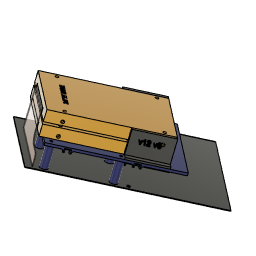
IDE Drive Bench Large and Models v12 v7 (Autodesk Fusion 360 design; units mm, degrees)
Autodesk Fusion 360 part; units mm, degrees
note: some values were not read from the file. Set by a fixed rule: which sketch regions a step uses.
sketch "Sketch1" plane through (0, 0, 0) normal (0, 1, 0) x (1, 0, 0)
  line L0 (0, 0) -> (-110, 0)
  line L1 (-110, 0) -> (-110, -88)
  line L2 (-110, -88) -> (0, -88)
  line L3 (0, -88) -> (0, 0)
  dimension "d1" = 110
  dimension "d2" = 88
  constraint horizontal L0
  constraint vertical L1
  constraint horizontal L2
  constraint vertical L3
  constraint coincident L0.start L3.end
  measures "d1" distance of L0.start L0.end
  measures "d2" distance of L0.start L2.end
extrude "Extrude1" add sketch "Sketch1" along normal blind 2.25 makes body 1
sketch "Pillars to JM003A" plane through (0, 2.25, 0) normal (0, 1, 0) x (-1, 0, 0)
  line L0 (0, 88) -> (0, 0)
  line L1 (0, 0) -> (110, 0)
  line L2 (110, 0) -> (110, 88)
  line L3 (110, 88) -> (0, 88)
  line L4 (5.6675, 45.75) -> (59.1675, 45.75)
  line L5 (59.1675, 45.75) -> (59.1675, 82.75)
  line L6 (59.1675, 82.75) -> (5.6675, 82.75)
  line L7 (5.6675, 82.75) -> (5.6675, 45.75)
  circle A0 centre (59.1675, 45.75) radius 1.25
  circle A1 centre (59.1675, 82.75) radius 1.25
  circle A2 centre (5.6675, 82.75) radius 1.25
  circle A3 centre (5.6675, 45.75) radius 1.25
  circle A4 centre (59.1675, 45.75) radius 3.5
  circle A5 centre (5.6675, 45.75) radius 3.5
  circle A6 centre (59.1675, 82.75) radius 3.5
  circle A7 centre (5.6675, 82.75) radius 3.5
  dimension "d5" = 53.5
  dimension "d6" = 37
  dimension "d7" = 2.5
  dimension "d8" = 2.5
  dimension "d9" = 2.5
  dimension "d10" = 2.5
  dimension "d11" = 7
  dimension "d12" = 7
  dimension "d13" = 7
  dimension "d14" = 7
  dimension "d184" = 5.25
  constraint horizontal L4
  constraint vertical L5
  constraint horizontal L6
  constraint vertical L7
  constraint coincident L4.end L5.start
  constraint coincident L5.end L6.start
  constraint coincident L6.end L7.start
  constraint coincident L4.start L7.end
  constraint concentric A0 A4
  constraint concentric A3 A5
  constraint concentric A1 A6
  constraint concentric A2 A7
  measures "d5" distance of L4.start L4.end
  measures "d6" distance of L4.start L6.end
  measures "d7" diameter of A0
  measures "d8" diameter of A1
  measures "d9" diameter of A2
  measures "d10" diameter of A3
  measures "d11" diameter of A4
  measures "d12" diameter of A5
  measures "d13" diameter of A6
  measures "d14" diameter of A7
  measures "d184" distance of L3 L6.end
extrude "Extrude2" add sketch "Pillars to JM003A" along normal blind 19.5 contours L4 L7 A3 A5 | L4 L7 A3 A5 | L4 L5 A0 A4 | L4 L5 A0 A4 | L6 L7 A2 A7 | L6 L7 A2 A7 | L5 L6 A1 A6 | L5 L6 A1 A6 bodies 1
sketch "Sketch3" plane through (0, 2.25, 0) normal (0, 1, 0) x (-1, 0, 0)
  circle A0 centre (59.1675, 45.75) radius 3.5
  circle A1 centre (59.1675, 82.75) radius 3.5
  line L0 (0, 88) -> (0, 0)
  line L1 (0, 0) -> (110, 0)
  line L2 (110, 0) -> (110, 88)
  line L3 (110, 88) -> (0, 88)
  circle A2 centre (5.6675, 82.75) radius 3.5
  circle A3 centre (5.6675, 45.75) radius 3.5
  line L4 (75, 0) -> (73.5, 0)
  line L5 (73.5, 0) -> (73.5, 2.5)
  line L6 (73.5, 2.5) -> (75, 2.5)
  line L7 (75, 2.5) -> (75, 0)
  line L8 (14.9953, 0) -> (16.4953, 0)
  line L9 (16.4953, 0) -> (16.4953, 2.5)
  line L10 (16.4953, 2.5) -> (14.9953, 2.5)
  line L11 (14.9953, 2.5) -> (14.9953, 0)
  line L12 (75, 88) -> (73.5, 88)
  line L13 (73.5, 88) -> (73.5, 85.5)
  line L14 (73.5, 85.5) -> (75, 85.5)
  line L15 (75, 85.5) -> (75, 88)
  line L16 (14.9794, 88) -> (16.4794, 88)
  line L17 (16.4794, 88) -> (16.4794, 85.5)
  line L18 (16.4794, 85.5) -> (14.9794, 85.5)
  line L19 (14.9794, 85.5) -> (14.9794, 88)
  line L20 (70, 0) -> (68.5, 0)
  line L21 (68.5, 0) -> (68.5, 2.5)
  line L22 (68.5, 2.5) -> (70, 2.5)
  line L23 (70, 2.5) -> (70, 0)
  line L24 (19.9953, 0) -> (21.4953, 0)
  line L25 (21.4953, 0) -> (21.4953, 2.5)
  line L26 (21.4953, 2.5) -> (19.9953, 2.5)
  line L27 (19.9953, 2.5) -> (19.9953, 0)
  line L28 (70, 88) -> (68.5, 88)
  line L29 (68.5, 88) -> (68.5, 85.5)
  line L30 (68.5, 85.5) -> (70, 85.5)
  line L31 (70, 85.5) -> (70, 88)
  line L32 (19.9794, 88) -> (21.4794, 88)
  line L33 (21.4794, 88) -> (21.4794, 85.5)
  line L34 (21.4794, 85.5) -> (19.9794, 85.5)
  line L35 (19.9794, 85.5) -> (19.9794, 88)
  dimension "d17" = 1.5
  dimension "d18" = 2.5
  dimension "d19" = 1.5
  dimension "d20" = 2.5
  dimension "d21" = 1.5
  dimension "d22" = 2.5
  dimension "d23" = 1.5
  dimension "d24" = 2.5
  dimension "d25" = 1.5
  dimension "d26" = 2.5
  dimension "d27" = 3.5
  dimension "d28" = 1.5
  dimension "d29" = 2.5
  dimension "d30" = 3.5
  dimension "d31" = 1.5
  dimension "d32" = 2.5
  dimension "d33" = 3.5
  dimension "d34" = 1.5
  dimension "d35" = 2.5
  dimension "d36" = 3.5
  dimension "d185" = 35
  dimension "d186" = 35
  constraint horizontal L4
  constraint vertical L5
  constraint horizontal L6
  constraint vertical L7
  constraint coincident L1 L4.start
  constraint horizontal L8
  constraint vertical L9
  constraint horizontal L10
  constraint vertical L11
  constraint coincident L1 L8.start
  constraint horizontal L12
  constraint vertical L13
  constraint horizontal L14
  constraint vertical L15
  constraint coincident L3 L12.start
  constraint horizontal L16
  constraint vertical L17
  constraint horizontal L18
  constraint vertical L19
  constraint coincident L3 L16.start
  constraint horizontal L20
  constraint vertical L21
  constraint horizontal L22
  constraint vertical L23
  constraint coincident L1 L20.start
  constraint horizontal L24
  constraint vertical L25
  constraint horizontal L26
  constraint vertical L27
  constraint coincident L1 L24.start
  constraint horizontal L28
  constraint vertical L29
  constraint horizontal L30
  constraint vertical L31
  constraint coincident L3 L28.start
  constraint horizontal L32
  constraint vertical L33
  constraint horizontal L34
  constraint vertical L35
  constraint coincident L3 L32.start
  measures "d17" distance of L4.start L4.end
  measures "d18" distance of L4.start L6.end
  measures "d19" distance of L8.start L8.end
  measures "d20" distance of L8.start L10.end
  measures "d21" distance of L12.start L12.end
  measures "d22" distance of L12.start L14.end
  measures "d23" distance of L16.start L16.end
  measures "d24" distance of L16.start L18.end
  measures "d25" distance of L20.start L20.end
  measures "d26" distance of L20.start L22.end
  measures "d27" distance of L5 L23
  measures "d28" distance of L24.start L24.end
  measures "d29" distance of L24.start L26.end
  measures "d30" distance of L9 L27
  measures "d31" distance of L28.start L28.end
  measures "d32" distance of L28.start L30.end
  measures "d33" distance of L13 L31
  measures "d34" distance of L32.start L32.end
  measures "d35" distance of L32.start L34.end
  measures "d36" distance of L17 L35
  measures "d185" distance of L2 L15
  measures "d186" distance of L2 L7
extrude "Extrude3" add sketch "Sketch3" along normal blind 2.5 contours L3 L16 L17 L18 L19 | L3 L32 L33 L34 L35 bodies 1
extrude "Extrude4" add sketch "Sketch3" along normal blind 2.5 contours L3 L28 L29 L30 L31 | L3 L12 L13 L14 L15 bodies 1
extrude "Extrude5" add sketch "Sketch3" along normal blind 2.5 contours L1 L20 L21 L22 L23 | L1 L4 L5 L6 L7 bodies 1
extrude "Extrude6" add sketch "Sketch3" along normal blind 2.5 contours L1 L8 L9 L10 L11 | L1 L24 L25 L26 L27 bodies 1
fillet "Fillet1" radius 1 2 edges at (-73.5, 3.5, 88) (-70, 3.5, 88) on bodies 1
fillet "Fillet2" radius 1 2 edges at (-19.9794, 3.5, 88) (-16.4794, 3.5, 88) on bodies 1
fillet "Fillet3" radius 1 2 edges at (-16.4953, 3.5, 0) (-19.9953, 3.5, 0) on bodies 1
fillet "Fillet4" radius 1 2 edges at (-70, 3.5, 0) (-73.5, 3.5, 0) on bodies 1
fillet "Fillet5" radius 2 4 edges at (-75, 2.25, 86.75) (-75, 2.25, 1.25) (-21.4953, 2.25, 1.25) (-21.4794, 2.25, 86.75) on bodies 1
fillet "Fillet6" radius 2 4 edges at (-21.7453, 2.25, 2.5) (-75.25, 2.25, 2.5) (-75.25, 2.25, 85.5) (-21.7294, 2.25, 85.5) on bodies 1
fillet "Fillet7" radius 2 4 edges at (-68.5, 2.25, 86.75) (-68.5, 2.25, 1.25) (-14.9794, 2.25, 86.75) (-14.9953, 2.25, 1.25) on bodies 1
fillet "Fillet8" radius 2 4 edges at (-68.25, 2.25, 2.5) (-14.7453, 2.25, 2.5) (-14.7294, 2.25, 85.5) (-68.25, 2.25, 85.5) on bodies 1
fillet "Fillet10" radius 1 4 edges at (-71.75, 2.25, 0) (-18.2453, 2.25, 0) (-18.2294, 2.25, 88) (-71.75, 2.25, 88) on bodies 1
sketch "Version String" plane through (0, 2.25, 0) normal (0, 1, 0) x (-1, 0, 0)
  line L0 (73.5, 87) -> (70, 87)
  line L1 (70, 87) -> (70, 83.5)
  line L2 (66.5, 83.5) -> (66.5, 88)
  line L3 (66.5, 88) -> (23.4794, 88)
  line L4 (23.4794, 88) -> (23.4794, 83.5)
  line L5 (23.4794, 83.5) -> (19.9794, 83.5)
  line L6 (19.9794, 83.5) -> (19.9794, 87)
  line L7 (19.9794, 87) -> (16.4794, 87)
  line L8 (16.4794, 87) -> (16.4794, 83.5)
  line L9 (16.4794, 83.5) -> (12.9794, 83.5)
  line L10 (12.9794, 83.5) -> (12.9794, 88)
  line L11 (12.9794, 88) -> (0, 88)
  line L12 (0, 88) -> (0, 0)
  line L13 (0, 0) -> (12.9953, 0)
  line L14 (12.9953, 0) -> (12.9953, 4.5)
  line L15 (12.9953, 4.5) -> (16.4953, 4.5)
  line L16 (16.4953, 4.5) -> (16.4953, 1)
  line L17 (16.4953, 1) -> (19.9953, 1)
  line L18 (19.9953, 1) -> (19.9953, 4.5)
  line L19 (19.9953, 4.5) -> (23.4953, 4.5)
  line L20 (23.4953, 4.5) -> (23.4953, 0)
  line L21 (23.4953, 0) -> (66.5, 0)
  line L22 (66.5, 0) -> (66.5, 4.5)
  line L23 (66.5, 4.5) -> (70, 4.5)
  line L24 (70, 4.5) -> (70, 1)
  line L25 (70, 1) -> (73.5, 1)
  line L26 (73.5, 1) -> (73.5, 4.5)
  line L27 (73.5, 4.5) -> (77, 4.5)
  line L28 (77, 4.5) -> (77, 0)
  line L29 (77, 0) -> (110, 0)
  line L30 (110, 0) -> (110, 88)
  line L31 (110, 88) -> (77, 88)
  line L32 (77, 88) -> (77, 83.5)
  line L33 (77, 83.5) -> (73.5, 83.5)
  line L34 (73.5, 83.5) -> (73.5, 87)
  line L35 (63.5441, 32.548) -> (63.5441, 16.8859) construction
  line L36 (63.5441, 16.8859) -> (69.5441, 16.8859) construction
  line L37 (69.5441, 16.8859) -> (69.5441, 32.548) construction
  line L38 (69.5441, 32.548) -> (63.5441, 32.548) construction
  circle A0 centre (5.6675, 82.75) radius 3.5
  circle A1 centre (5.6675, 45.75) radius 3.5
  circle A2 centre (59.1675, 45.75) radius 3.5
  line L39 (70, 83.5) -> (66.5, 83.5)
  circle A3 centre (59.1675, 82.75) radius 3.5
  text T0 "v12v3" font "Arial" height 6 align ink ink in box 0 x 0 at (63.5641, 32.538) x (0, -1) y (1, 0) spacing 1 height is em
  constraint perpendicular L35 L36
  constraint parallel L35 L37
  constraint parallel L36 L38
extrude "Extrude7" add sketch "Version String" along normal blind 1 text T0 bodies 1
fillet "Fillet11" radius 1 4 edges at (-4.5021, 21.75, 46.202) (-4.5021, 21.75, 83.202) (-58.0021, 21.75, 83.202) (-58.0021, 21.75, 46.202) on bodies 1
ref_plane "WorkPlane1" through (-55, -10, 44) normal (0, 1, 0) x (1, 0, 0)
sketch "Sketch5" plane through (0, 0, 0) normal (0, 1, 0) x (1, 0, 0)
sketch "Sketch6" plane through (-42.5, -10, 44) normal (0, 1, 0) x (1, 0, 0)
  line L0 (40.0162, -34.9034) -> (-59.9838, -34.9034)
  line L1 (-59.9838, -34.9034) -> (-59.9838, 35.0966)
  line L2 (-59.9838, 35.0966) -> (40.0162, 35.0966)
  line L3 (40.0162, 35.0966) -> (40.0162, -34.9034)
  dimension "d59" = 100
  dimension "d60" = 70
  constraint horizontal L0
  constraint vertical L1
  constraint horizontal L2
  constraint vertical L3
  measures "d59" distance of L0.start L0.end
  measures "d60" distance of L0.start L2.end
extrude "Extrude8" add sketch "Sketch6" against normal blind 10 separate body makes body 2
sketch "Sketch7" plane through (0, -20, 0) normal (0, -1, 0) x (1, 0, 0)
  line L0 (-102.4838, 8.9034) -> (-2.4838, 8.9034)
  line L1 (-2.4838, 8.9034) -> (-2.4838, 78.9034)
  line L2 (-2.4838, 78.9034) -> (-102.4838, 78.9034)
  line L3 (-102.4838, 78.9034) -> (-102.4838, 8.9034)
  line L4 (-20.7994, 59.6561) -> (-20.7994, 27.1781) construction
  line L5 (-20.7994, 27.1781) -> (-15.7994, 27.1781) construction
  line L6 (-15.7994, 27.1781) -> (-15.7994, 59.6561) construction
  line L7 (-15.7994, 59.6561) -> (-20.7994, 59.6561) construction
  text T0 "2.5\" FF DRIVE" font "Arial" height 5 align ink ink in box 0 x 0 at (-20.7794, 59.6461) x (0, -1) y (1, 0) spacing 1 height is em
  constraint perpendicular L4 L5
  constraint parallel L4 L6
  constraint parallel L5 L7
extrude "Extrude9" cut sketch "Sketch7" against normal blind 1 text T0 bodies 2
sketch "Sketch8" plane through (0, 0, 78.9034) normal (0, 0, 1) x (1, 0, 0)
  line L0 (-2.4838, -10) -> (-102.4838, -10)
  line L1 (-102.4838, -10) -> (-102.4838, -20)
  line L2 (-102.4838, -20) -> (-2.4838, -20)
  line L3 (-2.4838, -20) -> (-2.4838, -10)
  circle A0 centre (-16.4838, -13) radius 1.5
  line L4 (-2.4838, -10) -> (-102.4838, -10)
  circle A1 centre (-93.0838, -12.9925) radius 1.5
  dimension "d65" = 3
  dimension "d66" = 14
  dimension "d67" = 3
  dimension "d68" = 3
  dimension "d69" = 90.6
  measures "d65" diameter of A0
  measures "d66" distance of L3 A0.centre
  measures "d67" distance of A0.centre L4
  measures "d68" diameter of A1
  measures "d69" distance of L3 A1.centre
extrude "Extrude10" cut sketch "Sketch8" against normal blind 70 contours A1 bodies 2
extrude "Extrude11" cut sketch "Sketch8" against normal blind 70 contours A0 bodies 2
sketch "Sketch9" plane through (0, -10, 0) normal (0, 1, 0) x (-1, 0, 0)
  line L0 (2.4838, 8.9034) -> (102.4838, 8.9034)
  line L1 (102.4838, 8.9034) -> (102.4838, 78.9034)
  line L2 (102.4838, 78.9034) -> (2.4838, 78.9034)
  line L3 (2.4838, 78.9034) -> (2.4838, 8.9034)
  circle A0 centre (16.4838, 74.8334) radius 1.5
  line L4 (2.4838, 78.9034) -> (102.4838, 78.9034)
  circle A1 centre (16.4838, 12.9734) radius 1.5
  circle A2 centre (93.0838, 74.8334) radius 1.5
  circle A3 centre (93.0838, 12.9734) radius 1.5
  dimension "d74" = 3
  dimension "d75" = 14
  dimension "d76" = 4.07
  dimension "d77" = 3
  dimension "d78" = 14
  dimension "d79" = 4.07
  dimension "d80" = 3
  dimension "d81" = 90.6
  dimension "d82" = 4.07
  dimension "d83" = 3
  dimension "d84" = 90.6
  dimension "d85" = 4.07
  measures "d74" diameter of A0
  measures "d75" distance of L3 A0.centre
  measures "d76" distance of A0.centre L4
  measures "d77" diameter of A1
  measures "d78" distance of L3 A1.centre
  measures "d79" distance of L0 A1.centre
  measures "d80" diameter of A2
  measures "d81" distance of L3 A2.centre
  measures "d82" distance of L2 A2.centre
  measures "d83" diameter of A3
  measures "d84" distance of L3 A3.centre
  measures "d85" distance of L0 A3.centre
extrude "Extrude12" cut sketch "Sketch9" against normal blind 10 contours A0 | A1 | A2 | A3 bodies 2
sketch "IDE Connector Recess" plane through (-2.4838, 0, 0) normal (1, 0, 0) x (0, 0, -1)
  line L0 (-8.9034, -10) -> (-78.9034, -10)
  line L1 (-78.9034, -10) -> (-78.9034, -20)
  line L2 (-78.9034, -20) -> (-8.9034, -20)
  line L3 (-8.9034, -20) -> (-8.9034, -10)
  line L4 (-62.9034, -10) -> (-18.9034, -10)
  line L5 (-18.9034, -10) -> (-18.9034, -14)
  line L6 (-18.9034, -14) -> (-62.9034, -14)
  line L7 (-62.9034, -14) -> (-62.9034, -10)
  dimension "d100" = 44
  dimension "d101" = 4
  dimension "d174" = 16
  dimension "d175" = 10
  constraint horizontal L4
  constraint vertical L5
  constraint horizontal L6
  constraint vertical L7
  constraint coincident L0 L4.start
  measures "d100" distance of L4.start L4.end
  measures "d101" distance of L4.start L6.end
  measures "d174" distance of L1 L7
  measures "d175" distance of L3 L5
extrude "Extrude13" cut sketch "IDE Connector Recess" against normal blind 4 contours L0 L4 L5 L6 L7 bodies 2
sketch "Sketch11" plane through (0, 0, 0) normal (0, -1, 0) x (1, 0, 0)
  line L0 (0, 0) -> (0, 88)
  line L1 (0, 88) -> (-110, 88)
  line L2 (-110, 88) -> (-110, 0)
  line L3 (-110, 0) -> (0, 0)
  line L4 (-0.0039, 28.8454) -> (-4.0039, 28.8454)
  line L5 (-4.0039, 28.8454) -> (-4.0039, 72.8454)
  line L6 (-4.0039, 72.8454) -> (-0.0039, 72.8454)
  line L7 (-0.0039, 72.8454) -> (-0.0039, 28.8454)
  dimension "d104" = 4
  dimension "d105" = 44
  constraint horizontal L4
  constraint vertical L5
  constraint horizontal L6
  constraint vertical L7
  measures "d104" distance of L4.start L4.end
  measures "d105" distance of L4.start L6.end
sketch "Sketch12" plane through (0, 0, 0) normal (0, 1, 0) x (1, 0, 0)
  line L0 (15.0376, -24.9871) -> (11.0376, -24.9871)
  line L1 (11.0376, -24.9871) -> (11.0376, -68.9871)
  line L2 (11.0376, -68.9871) -> (15.0376, -68.9871)
  line L3 (15.0376, -68.9871) -> (15.0376, -24.9871)
  dimension "d106" = 4
  dimension "d107" = 44
  constraint horizontal L0
  constraint vertical L1
  constraint horizontal L2
  constraint vertical L3
  measures "d106" distance of L0.start L0.end
  measures "d107" distance of L0.start L2.end
extrude "Extrude14" add sketch "Sketch12" along normal blind 4 separate body makes body 3
move_body "Move1" bodies 3 to x (1, 0, 0) y (0, 1, 0) z (0, 0, 1) at (-17.4241, -4.5506, 3.881)
copy_body "CopyPasteBodies1" bodies 3 makes body 4
move_body "Move2" bodies 4 to x (1, 0, 0) y (0, 1, 0) z (0, 0, 1) at (0, -5.6283, 0)
move_body "Move3" bodies 2 to x (1, 0, 0) y (0, 1, 0) z (0, 0, 1) at (0, -7.1851, -0.2395)
ref_plane "WorkPlane2" through (-5.6675, 31.75, 45.75) normal (0, 1, 0) x (-1, 0, 0)
sketch "JM003A Card Outlone" plane through (-5.6675, 31.75, 44.8014) normal (0, 1, 0) x (1, 0, 0)
  line L0 (16.3291, -49.8685) -> (-141.6709, -49.8685)
  line L1 (-141.6709, -49.8685) -> (-141.6709, 40.1315)
  line L2 (-141.6709, 40.1315) -> (16.3291, 40.1315)
  line L3 (16.3291, 40.1315) -> (16.3291, -49.8685)
  line L4 (-45.6709, 40.1315) -> (-141.6709, 40.1315)
  line L5 (-141.6709, 40.1315) -> (-141.6709, 73.6737)
  line L6 (-141.6709, 73.6737) -> (-45.6709, 73.6737)
  line L7 (-45.6709, 73.6737) -> (-45.6709, 40.1315)
  dimension "d111" = 158
  dimension "d112" = 90
  dimension "d113" = 96
  dimension "d114" = 62
  constraint horizontal L0
  constraint vertical L1
  constraint horizontal L2
  constraint vertical L3
  constraint horizontal L4
  constraint vertical L5
  constraint horizontal L6
  constraint vertical L7
  constraint coincident L2 L4.start
  measures "d111" distance of L0.start L0.end
  measures "d112" distance of L0.start L2.end
  measures "d113" distance of L5.end L6.end
  measures "d114" distance of L3 L7
extrude "Extrude15" add sketch "JM003A Card Outlone" along normal blind 0.6 separate body makes body 5
sketch "Sketch15" plane through (0, 32.35, 0) normal (0, 1, 0) x (-1, 0, 0)
  line L0 (51.3384, -28.8723) -> (147.3384, -28.8723)
  line L1 (147.3384, -28.8723) -> (147.3384, 94.6698)
  line L2 (147.3384, 94.6698) -> (-10.6616, 94.6698)
  line L3 (-10.6616, 94.6698) -> (-10.6616, 4.6698)
  line L4 (-10.6616, 4.6698) -> (51.3384, 4.6698)
  line L5 (51.3384, 4.6698) -> (51.3384, -28.8723)
  circle A0 centre (4.3384, 89.6698) radius 1.5
  circle A1 centre (4.3384, 50.6698) radius 1.5
  circle A2 centre (69.3384, 50.6698) radius 1.5
  circle A3 centre (69.3384, 89.6698) radius 1.5
  dimension "d121" = 3
  dimension "d122" = 15
  dimension "d123" = 5
  dimension "d124" = 3
  dimension "d125" = 15
  dimension "d126" = 39
  dimension "d127" = 3
  dimension "d128" = 80
  dimension "d129" = 3
  dimension "d130" = 5
  dimension "d131" = 39
  dimension "d134" = 80
  measures "d121" diameter of A0
  measures "d122" distance of L3 A0.centre
  measures "d123" distance of L2 A0.centre
  measures "d124" diameter of A1
  measures "d125" distance of L3 A1.centre
  measures "d126" distance of A0.centre A1.centre
  measures "d127" diameter of A2
  measures "d128" distance of L3 A2.centre
  measures "d129" diameter of A3
  measures "d130" distance of L2 A3.centre
  measures "d131" vertical distance of A2.centre A3.centre
  measures "d134" distance of L3 A3.centre
extrude "Extrude16" cut sketch "Sketch15" against normal blind 7 contours A0 | A1 | A2 | A3 bodies 5
hole "Hole5" at (-5.6573, 0, 45.7372) direction (0, 1, 0) diameter 2.5 depth 25 tip angle 118 bodies 1
hole "Hole6" at (-5.6635, 0, 82.7531) direction (0, 1, 0) diameter 2.5 depth 25 tip angle 118 bodies 1
hole "Hole7" at (-59.1675, 2.25, 82.75) direction (0, -1, 0) diameter 2.5 depth 25 tip angle 118 bodies 1
hole "Hole8" at (-59.1675, 2.25, 45.75) direction (0, -1, 0) diameter 2.5 depth 25 tip angle 118 bodies 1
copy_body "CopyPasteBodies4" bodies 2 makes body 6
move_body "Move6" bodies 6 to x (1, 0, 0) y (0, 1, 0) z (0, 0, 1) at (0, -15, 0)
move_body "Move7" bodies 5 to x (1, 0, 0) y (0, 1, 0) z (0, 0, 1) at (0, -10, 0)
move_body "Move8" bodies 5 to x (1, 0, 0) y (0, 1, 0) z (0, 0, 1) at (-1.3137, 0, -5.821)
sketch "IDE44 Male on JM003A" plane through (0, 21.75, 0) normal (0, -1, 0) x (1, 0, 0)
  circle A0 centre (-70.6521, 44.8488) radius 1.5
  circle A1 centre (-5.6521, 44.8488) radius 1.5
  circle A2 centre (-70.6521, 83.8488) radius 1.5
  circle A3 centre (-5.6521, 83.8488) radius 1.5
  line L0 (-148.6521, -34.6933) -> (-52.6521, -34.6933)
  line L1 (-52.6521, -34.6933) -> (-52.6521, -1.1512)
  line L2 (-52.6521, -1.1512) -> (9.3479, -1.1512)
  line L3 (9.3479, -1.1512) -> (9.3479, 88.8488)
  line L4 (9.3479, 88.8488) -> (-148.6521, 88.8488)
  line L5 (-148.6521, 88.8488) -> (-148.6521, -34.6933)
  line L6 (2.3479, 86.8488) -> (6.3479, 86.8488)
  line L7 (6.3479, 86.8488) -> (6.3479, 42.8488)
  line L8 (6.3479, 42.8488) -> (2.3479, 42.8488)
  line L9 (2.3479, 42.8488) -> (2.3479, 86.8488)
  dimension "d147" = 4
  dimension "d148" = 44
  dimension "d149" = 3
  dimension "d150" = 2
  constraint horizontal L6
  constraint vertical L7
  constraint horizontal L8
  constraint vertical L9
  measures "d147" distance of L6.start L6.end
  measures "d148" distance of L6.start L8.end
  measures "d149" distance of L3 L7
  measures "d150" distance of L4 L6
move_body "Move9" bodies 2 to x (1, 0, 0) y (0, 1, 0) z (0, 0, 1) at (0, 17, 0)
move_body "Move10" bodies 3 to x (1, 0, 0) y (0, 1, 0) z (0, 0, 1) at (6, 0, 0)
move_body "Move11" bodies 2 to x (1, 0, 0) y (0, 1, 0) z (0, 0, 1) at (6, 0, 0)
hole "Hole9" at (-10.4584, 2.25, 74.622) direction (0, -1, 0) diameter 3 depth 25 tip angle 118 bodies 1 2
hole "Hole10" at (-87.1052, 2.25, 74.5527) direction (0, -1, 0) diameter 3 depth 25 tip angle 118 bodies 1 2
hole "Hole11" at (-10.5018, 2.25, 12.7427) direction (0, -1, 0) diameter 3 depth 25 tip angle 118 bodies 1 2
hole "Hole12" at (-87.1019, 2.25, 12.7339) direction (0, -1, 0) diameter 3 depth 25 tip angle 118 bodies 1 2
move_body "Move12" bodies 6 to x (1, 0, 0) y (0, 1, 0) z (0, 0, 1) at (6, 20, 0)
move_body "Move13" bodies 4 to x (1, 0, 0) y (0, 1, 0) z (0, 0, 1) at (6, 0, 0)
move_body "Move14" bodies 4 to x (1, 0, 0) y (0, 1, 0) z (0, 0, 1) at (0, -6, 0)
move_body "Move15" bodies 4 to x (1, 0, 0) y (0, 1, 0) z (0, 0, 1) at (0, 0, -0.2)
move_body "Move16" bodies 3 to x (1, 0, 0) y (0, 1, 0) z (0, 0, 1) at (0, 0.1, 0)
move_body "Move17" bodies 3 to x (1, 0, 0) y (0, 1, 0) z (0, 0, 1) at (0, 0.27, -0.25)
ref_plane "WorkPlane3" through (3.6135, -14.1789, 50.6681) normal (1, 0, 0) x (0, 0, -1)
sketch "IDE44 Riser Board" plane through (3.6135, -14.1789, 50.6681) normal (1, 0, 0) x (0, 0, -1)
  line L0 (32.2, -0.4211) -> (-37.8, -0.4211)
  line L1 (-37.8, -0.4211) -> (-37.8, 34.8289)
  line L2 (-37.8, 34.8289) -> (32.2, 34.8289)
  line L3 (32.2, 34.8289) -> (32.2, -0.4211)
  line L4 (51.8193, 35.9289) -> (-38.1807, 35.9289)
  line L5 (-22, -2) -> (-22, 2)
  line L6 (-21.95, 9.9983) -> (-21.95, 13.9983)
  dimension "d166" = 1.1
  dimension "d167" = 35.25
  dimension "d168" = 70
  constraint horizontal L0
  constraint vertical L1
  constraint horizontal L2
  constraint vertical L3
  measures "d166" distance of L2 L4
  measures "d167" distance of L0 L2
  measures "d168" distance of L1 L3
extrude "Extrude17" add sketch "IDE44 Riser Board" along normal blind 0.6 separate body makes body 7
sketch "IDE44 Riser Board Cutout" plane through (4.2135, 0, 0) normal (1, 0, 0) x (0, 0, -1)
  line L0 (-18.4681, 20.65) -> (-88.4681, 20.65)
  line L1 (-88.4681, 20.65) -> (-88.4681, -14.6)
  line L2 (-88.4681, -14.6) -> (-18.4681, -14.6)
  line L3 (-18.4681, -14.6) -> (-18.4681, 20.65)
  line L4 (-62.9681, -14.6) -> (-88.4681, -14.6)
  line L5 (-88.4681, -14.6) -> (-88.4681, 10.4)
  line L6 (-88.4681, 10.4) -> (-62.9681, 10.4)
  line L7 (-62.9681, 10.4) -> (-62.9681, -14.6)
  arc A0 (-88.4681, 14.689) -> (-83.0243, 10.4) centre (-84.0567, 14.689) ccw
  arc A1 (-62.9681, 1.0363) -> (-71.052, 10.4) centre (-71.3823, 1.9435) ccw
  line L8 (-62.6639, -0.1851) -> (-18.6639, -0.1851)
  line L9 (-88.4681, 20.65) -> (-18.4681, 20.65)
  line L10 (-62.6639, -12.1851) -> (-18.6639, -12.1851)
  line L11 (-18.4681, -14.6) -> (-88.4681, -14.6)
  dimension "d173" = 25
  dimension "d176" = 25.5
  dimension "d177" = 44.5
  dimension "d182" = 19.3351
  dimension "d183" = 3.9149
  constraint horizontal L4
  constraint vertical L5
  constraint horizontal L6
  constraint vertical L7
  constraint coincident L1 L5.end
  constraint coincident L2 L4.start
  constraint tangent L1 A0
  constraint coincident L1 A0.start
  constraint coincident L6 A0.end
  constraint coincident L7 A1.start
  constraint coincident L6 A1.end
  measures "d173" distance of L4 L6
  measures "d176" distance of L5 L7
  measures "d177" distance of L3 L7
extrude "Extrude20" cut sketch "IDE44 Riser Board Cutout" against normal blind 0.6 contours L1 L6 A0 | L1 L2 L4 L5 L6 L7 A0 A1 L11 | L6 A0 bodies 7
move_body "Move18" bodies 3 to x (1, 0, 0) y (0, 1, 0) z (0, 0, 1) at (0, 0, -10)
move_body "Move19" bodies 4 to x (1, 0, 0) y (0, 1, 0) z (0, 0, 1) at (0, 0, -10)
sketch "Sketch19" plane through (0, 0, 0) normal (0, -1, 0) x (1, 0, 0)
  circle A0 centre (-87.1019, 12.7339) radius 1.5
  circle A1 centre (-10.5018, 12.7427) radius 1.5
  circle A2 centre (-87.1052, 74.5527) radius 1.5
  circle A3 centre (-10.4584, 74.622) radius 1.5
  circle A4 centre (-59.1675, 45.75) radius 1.25
  circle A5 centre (-59.1675, 82.75) radius 1.25
  circle A6 centre (-5.6635, 82.7531) radius 1.25
  circle A7 centre (-5.6573, 45.7372) radius 1.25
  line L0 (0, 0) -> (0, 88)
  line L1 (0, 88) -> (-110, 88)
  line L2 (-110, 88) -> (-110, 0)
  line L3 (-110, 0) -> (0, 0)
ref_plane "WorkPlane4" through (-96.4838, -17.1851, 43.6639) normal (-1, 0, 0) x (0, 0, -1)
sketch "Sketch20" plane through (-96.4838, -17.1851, 43.6639) normal (-1, 0, 0) x (0, 0, -1)
  line L0 (-35.001, 5.0042) -> (-38.001, 5.0042)
  line L1 (-38.001, 5.0042) -> (-38.001, -18.9958)
  line L2 (-38.001, -18.9958) -> (-35.001, -18.9958)
  line L3 (-35.001, -18.9958) -> (-35.001, 5.0042)
  line L4 (35.001, 5.0042) -> (38.001, 5.0042)
  line L5 (38.001, 5.0042) -> (38.001, -18.9958)
  line L6 (38.001, -18.9958) -> (35.001, -18.9958)
  line L7 (35.001, -18.9958) -> (35.001, 5.0042)
  line L8 (-35, -5) -> (-35, 5)
  line L9 (35, -5) -> (35, 5)
  line L10 (-35.001, -5.1732) -> (35.001, -5.1732)
  line L11 (35.001, -5.1732) -> (35.001, -6.7968)
  line L12 (35.001, -6.7968) -> (-35.001, -6.7968)
  line L13 (-35.001, -6.7968) -> (-35.001, -5.1732)
  line L14 (38.001, -18.9958) -> (43.001, -18.9958)
  line L15 (43.001, -18.9958) -> (43.001, -15.9958)
  line L16 (43.001, -15.9958) -> (38.001, -15.9958)
  line L17 (38.001, -15.9958) -> (38.001, -18.9958)
  line L18 (-38.001, -18.9958) -> (-43.001, -18.9958)
  line L19 (-43.001, -18.9958) -> (-43.001, -15.9958)
  line L20 (-43.001, -15.9958) -> (-38.001, -15.9958)
  line L21 (-38.001, -15.9958) -> (-38.001, -18.9958)
  dimension "d188" = 3
  dimension "d189" = 24
  dimension "d190" = 3
  dimension "d191" = 24
  dimension "d192" = 0.001
  dimension "d193" = 0.001
  dimension "d209" = 5
  dimension "d210" = 3
  dimension "d211" = 5
  dimension "d212" = 3
  constraint horizontal L0
  constraint vertical L1
  constraint horizontal L2
  constraint vertical L3
  constraint horizontal L4
  constraint vertical L5
  constraint horizontal L6
  constraint vertical L7
  constraint horizontal L10
  constraint vertical L11
  constraint horizontal L12
  constraint vertical L13
  constraint coincident L7 L11.end
  constraint coincident L3 L10.start
  constraint horizontal L14
  constraint vertical L15
  constraint horizontal L16
  constraint vertical L17
  constraint horizontal L18
  constraint vertical L19
  constraint horizontal L20
  constraint vertical L21
  measures "d188" distance of L0.start L0.end
  measures "d189" distance of L0.start L2.end
  measures "d190" distance of L4.start L4.end
  measures "d191" distance of L4.start L6.end
  measures "d192" distance of L3 L8
  measures "d193" distance of L7 L9
  measures "d209" distance of L5.end L14.end
  measures "d210" distance of L5.end L16.end
  measures "d211" distance of L1.end L18.end
  measures "d212" distance of L1.end L20.end
extrude "Extrude23" add sketch "Sketch20" along normal blind 35 separate body makes body 8
sketch "Sketch21" plane through (0, 0, 0) normal (0, -1, 0) x (1, 0, 0)
  circle A0 centre (-87.1019, 12.7339) radius 1.5
  circle A1 centre (-10.5018, 12.7427) radius 1.5
  circle A2 centre (-87.1052, 74.5527) radius 1.5
  circle A3 centre (-10.4584, 74.622) radius 1.5
  circle A4 centre (-59.1675, 45.75) radius 1.25
  circle A5 centre (-59.1675, 82.75) radius 1.25
  circle A6 centre (-5.6635, 82.7531) radius 1.25
  circle A7 centre (-5.6573, 45.7372) radius 1.25
  line L0 (0, 0) -> (0, 88)
  line L1 (0, 88) -> (-110, 88)
  line L2 (-110, 88) -> (-110, 0)
  line L3 (-110, 0) -> (0, 0)
  circle A8 centre (-13.4584, 74.622) radius 1.5
  circle A9 centre (-90.1052, 74.5527) radius 1.5
  circle A10 centre (-90.1019, 12.7339) radius 1.5
  circle A11 centre (-13.5018, 12.7427) radius 1.5
  line L4 (-90.0922, 14.2338) -> (-87.1019, 14.2339)
  line L5 (-90.0922, 11.2339) -> (-87.1019, 11.2339)
  line L6 (-10.5167, 14.2339) -> (-13.4973, 14.2427)
  line L7 (-13.4973, 11.2428) -> (-10.5018, 11.2427)
  line L8 (-10.4584, 76.122) -> (-13.4584, 76.122)
  line L9 (-13.4584, 73.122) -> (-10.4584, 73.122)
  line L10 (-87.1035, 76.0527) -> (-90.1052, 76.0527)
  line L11 (-90.1052, 73.0527) -> (-87.1052, 73.0527)
  dimension "d199" = 3
  dimension "d200" = 3
  dimension "d201" = 3
  dimension "d202" = 3
  dimension "d203" = 3
  dimension "d204" = 3
  dimension "d205" = 3
  dimension "d206" = 3
  constraint coincident A10 L4.start
  constraint coincident A0 L4.end
  constraint tangent A0 L4
  constraint coincident A10 L5.start
  constraint coincident A0 L5.end
  constraint tangent A0 L5
  constraint coincident A11 L6.end
  constraint tangent A11 L6
  constraint coincident A11 L7.start
  constraint coincident A1 L7.end
  constraint tangent A1 L7
  constraint coincident A3 L8.start
  constraint coincident A8 L8.end
  constraint tangent A8 L8
  constraint parallel L3 L8
  constraint coincident A8 L9.start
  constraint coincident A3 L9.end
  constraint tangent A3 L9
  constraint parallel L8 L9
  constraint coincident A2 L10.start
  constraint coincident A9 L10.end
  constraint tangent A9 L10
  constraint coincident A9 L11.start
  constraint coincident A2 L11.end
  constraint tangent A2 L11
  constraint horizontal L11
  measures "d199" diameter of A8
  measures "d200" distance of A3.centre A8.centre
  measures "d201" diameter of A9
  measures "d202" distance of A2.centre A9.centre
  measures "d203" diameter of A10
  measures "d204" distance of A0.centre A10.centre
  measures "d205" diameter of A11
  measures "d206" distance of A1.centre A11.centre
extrude "Extrude22" cut sketch "Sketch21" against normal blind 5 contours A0 A10 L4 | A0 A10 L5 | A10 | A1 A11 L6 | A11 | A1 A11 L7 | A2 A9 L10 | A2 A9 L11 | A9 | A3 A8 L8 | A3 A8 L9 | A8 bodies 1
move_body "Move20" bodies 8 to x (1, 0, 0) y (0, 1, 0) z (0, 0, 1) at (35, 0, 0)
hole "Hole14" at (-87.062, -15.1805, 81.6649) direction (0, 0, -1) diameter 3 depth 1000 tip angle 118 bodies 6 8
sketch "Version ID" plane through (0, 0, 81.6649) normal (0, 0, 1) x (1, 0, 0)
  circle A0 centre (-87.062, -15.1805) radius 1.5
  line L0 (-61.4838, -22.1893) -> (-61.4838, -1.1893)
  line L1 (-61.4838, -1.1893) -> (-96.4838, -1.1893)
  line L2 (-96.4838, -1.1893) -> (-96.4838, -22.1893)
  line L3 (-96.4838, -22.1893) -> (-61.4838, -22.1893)
  line L4 (-68.4812, -12.142) -> (-85.8073, -12.142) construction
  line L5 (-85.8073, -12.142) -> (-85.8073, -18.142) construction
  line L6 (-85.8073, -18.142) -> (-68.4812, -18.142) construction
  line L7 (-68.4812, -18.142) -> (-68.4812, -12.142) construction
  text T0 "v12 v6" font "Arial" height 6 align ink ink in box 0 x 0 at (-68.4912, -12.162) x (-1, 0) y (0, -1) spacing 1 height is em
  constraint perpendicular L4 L5
  constraint parallel L4 L6
  constraint parallel L5 L7
extrude "Extrude24" add sketch "Version ID" along normal blind 2 text T0 bodies 8
move_face "OffsetFaces1" offset 1.5 2 faces at (-84.8171, 1.8107, 81.3316) (-84.8171, 1.8107, 3.3296) on bodies 8
named bodies: "Part", "2.5  Rotary Drive Master", "Master 798-A3D-44DA-2DSE71", "Slave 798-A3D-44DA-2DSE71", "JM003A", "2.5  Rotary Drive", "2.5  Rotary Drive Slave", "IDE44 Riser Board", "Dual Drive Separator"
